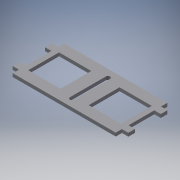
# Autodesk Inventor part: center mount
Saved by Autodesk Inventor 2016 (Build 200138000, 138)
## iProperties
Created: 2016-12-04
Part Number: center mount
Material: Generic
Document SubType Name: Modeling
Designer: William
Density: 1 g/cm^3
Appearance: Default
Author: William
Autodesk Inventor part; units mm, degrees
ref_plane "YZ Plane" through (0, 0, 0) normal (1, 0, 0) x (0, 1, 0)
ref_plane "XZ Plane" through (0, 0, 0) normal (0, 1, 0) x (-1, 0, 0)
ref_plane "XY Plane" through (0, 0, 0) normal (0, 0, 1) x (1, 0, 0)
sketch "Sketch1" plane through (0, 0, 0) normal (0, 0, 1) x (1, 0, 0)
  line L0 (0, 0) -> (180, 0)
  line L1 (180, 0) -> (180, 80)
  line L2 (180, 80) -> (0, 80)
  line L3 (0, 80) -> (0, 0)
  dimension "d0" = 180
  dimension "d1" = 80
  constraints: 8 end point, 2 parallel, 1 horizontal, 1 perpendicular
  measures "d0" distance of L1.end L2.end
  measures "d1" distance of L0.end L1.end
extrude "Extrusion1" add sketch "Sketch1" along normal blind 10.4
sketch "Sketch2" plane through (0, 0, 10.4) normal (0, 0, 1) x (1, 0, 0)
  line L0 (0, 80) -> (0, 0) projected
  line L1 (0, 60) -> (10, 60)
  line L2 (10, 60) -> (10, 20)
  line L3 (10, 20) -> (0, 20)
  line L4 (0, 9.6) -> (10, 9.6)
  line L5 (10, 9.6) -> (10, 0)
  line L6 (0, 0) -> (180, 0) projected
  line L7 (0, 70.4) -> (10, 70.4)
  line L8 (10, 70.4) -> (10, 80)
  line L9 (180, 80) -> (0, 80) projected
  line L10 (170, 80) -> (170, 70.4)
  line L11 (170, 70.4) -> (180, 70.4)
  line L12 (180, 0) -> (180, 80) projected
  line L13 (180, 60) -> (170, 60)
  line L14 (170, 60) -> (170, 20)
  line L15 (170, 20) -> (180, 20)
  line L16 (170, 0) -> (170, 9.6)
  line L17 (170, 9.6) -> (180, 9.6)
  line L18 (162, 64) -> (162, 16)
  line L19 (18, 16) -> (18, 64)
  line L20 (112, 64) -> (112, 16)
  line L21 (68, 16) -> (68, 64)
  line L22 (18, 64) -> (68, 64)
  line L23 (112, 64) -> (162, 64)
  line L24 (162, 16) -> (112, 16)
  line L25 (68, 16) -> (18, 16)
  line L26 (93.25, 12) -> (93.25, 68)
  line L27 (86.75, 12) -> (86.75, 68)
  arc A0 (86.75, 12) -> (93.25, 12) centre (90, 12) ccw
  arc A1 (93.25, 68) -> (86.75, 68) centre (90, 68) ccw
  dimension "d4" = 40
  dimension "d5" = 10.4
  dimension "d6" = 10.4
  dimension "d7" = 9.6
  dimension "d8" = 10
  dimension "d9" = 40
  dimension "d10" = 10.4
  dimension "d11" = 10.4
  dimension "d13" = 10
  dimension "d14" = 10
  dimension "d15" = 9.6
  dimension "d19" = 8
  dimension "d21" = 8
  dimension "d22" = 50
  dimension "d23" = 50
  dimension "d24" = 16
  dimension "d25" = 16
  dimension "d26" = 16
  dimension "d27" = 16
  dimension "d31" = 12
  dimension "d32" = 12
  dimension "d33" = 6.5
  dimension "d34" = 18.75
  constraints: 48 end point, 18 point on line, 9 perpendicular, 7 parallel, 4 horizontal, 4 point on circle, 4 tangent, 3 vertical, 2 centre point, 2 horizontal alignment
  measures "d4" distance between parallel lines of L3 L1
  measures "d5" distance between parallel lines of L1 L7
  measures "d6" distance between parallel lines of L3 L4
  measures "d7" distance of L7.end L8.end
  measures "d8" distance between parallel lines of L0 L2
  measures "d9" distance of L13.end L14.end
  measures "d10" distance between parallel lines of L13 L11
  measures "d11" distance between parallel lines of L17 L15
  measures "d13" distance between parallel lines of L14 L12
  measures "d14" distance between parallel lines of L12 L10
  measures "d15" distance of L16.start L16.end
  measures "d19" distance between parallel lines of L2 L19
  measures "d21" distance between parallel lines of L14 L18
  measures "d22" distance between parallel lines of L19 L21
  measures "d23" distance between parallel lines of L18 L20
  measures "d24" distance between parallel lines of L9 L22
  measures "d25" distance between parallel lines of L9 L23
  measures "d26" distance between parallel lines of L6 L24
  measures "d27" distance between parallel lines of L6 L25
  measures "d31" distance from line of L6 L26.start
  measures "d32" distance from line of L9 L26.end
  measures "d33" distance between parallel lines of L26 L27
  measures "d34" distance between parallel lines of L20 L26
extrude "Extrusion2" cut sketch "Sketch2" against normal up to next contours L9 L8 L7 L0 | L1 L2 L3 L0 | L9 L12 L11 L10 | L4 L5 L6 L0 | L12 L15 L14 L13 | L16 L17 L12 L6 | L18 L24 L20 L23 | L19 L22 L21 L25 | A0 L27 A1 L26
equation "\"d24\" = d26"
equation "\"d25\" = d26"
equation "\"d27\" = d26"
body "Solid1"
